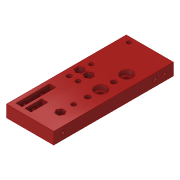
# Autodesk Inventor part: Coupler lift short left
Saved by Autodesk Inventor 2020 (Build 240168000, 168)
## iProperties
Created: 2019-10-02
Part Number: Coupler lift short left
Material: Generic
Document SubType Name: Modeling
Designer: ball
Density: 1 g/cm^3
Appearance: Default
Author: ball
Autodesk Inventor part; units mm, degrees
ref_plane "YZ Plane" through (0, 0, 0) normal (1, 0, 0) x (0, 1, 0)
sketch "Sketch1" plane through (0, 0, 0) normal (0, 1, 0) x (-1, 0, 0)
  line L0 (0, 0) -> (35.5, 0)
  line L1 (35.5, 0) -> (35.5, -90)
  line L2 (35.5, -90) -> (0, -90)
  line L3 (0, -90) -> (0, 0)
  dimension "d0" = 35.5
  dimension "d1" = 90
  constraints: 8 end point, 2 parallel, 1 horizontal, 1 perpendicular
  measures "d0" distance of L1.end L2.end
  measures "d1" distance of L0.end L1.end
extrude "BlockShape" add sketch "Sketch1" along normal blind 9
sketch "Sketch3" plane through (0, 0, 0) normal (0, -1, 0) x (1, 0, 0)
  circle A0 centre (-10, -25) radius 3.25 construction
  line L0 (0, 0) -> (-35.5, 0) projected
  line L1 (-35.5, 0) -> (-35.5, -90) projected
  line L2 (-11.6286, -27.8125) -> (-13.25, -24.9958)
  line L3 (-13.25, -24.9958) -> (-11.6214, -22.1833)
  line L4 (-11.6214, -22.1833) -> (-8.3714, -22.1875)
  line L5 (-8.3714, -22.1875) -> (-6.75, -25.0042)
  line L6 (-6.75, -25.0042) -> (-8.3786, -27.8167)
  line L7 (-8.3786, -27.8167) -> (-11.6286, -27.8125)
  line L8 (0, -90) -> (0, 0) projected
  dimension "d15" = 6.5
  dimension "d16" = 25
  dimension "d26" = 10
  constraints: 12 end point, 1 coincident, 16 other
  measures "d16" distance from line of L0 point (-10, -25)
  measures "d26" distance from line of L8 point (-10, -25)
extrude "SlideMountingNutWell1" cut sketch "Sketch3" against normal blind 5
sketch "Sketch5" plane through (0, 9, 0) normal (0, 1, 0) x (1, 0, 0)
  line L0 (0, 0) -> (0, 90) projected
  line L1 (-35.5, 0) -> (0, 0) projected
  circle A0 centre (-10, 25) radius 1.7
  circle A1 centre (-10, 15) radius 1.7
  dimension "d36" = 3.4
  dimension "d37" = 25
  dimension "d137" = 3.4
  dimension "d138" = 15
  constraints: 2 centre point
  measures "d36" diameter of A0
  measures "d37" distance from line of L1 A0.centre
  measures "d137" diameter of A1
  measures "d138" distance from line of L1 A1.centre
extrude "SlideMountingHoles" cut sketch "Sketch5" against normal through all
sketch "Sketch6" plane through (0, 9, 0) normal (0, 1, 0) x (1, 0, 0)
  line L0 (-32.5, 4) -> (-27.7502, 4)
  line L1 (-27.7502, 4) -> (-27.7502, 29.4)
  line L2 (-27.7502, 29.4) -> (-32.5, 29.4)
  line L3 (-32.5, 29.4) -> (-32.5, 4)
  line L4 (-35.5, 0) -> (0, 0) projected
  line L5 (-35.5, 90) -> (-35.5, 0) projected
  line L6 (-25.7502, 4) -> (-21.0002, 4)
  line L7 (-21.0002, 4) -> (-21.0002, 16.7)
  line L8 (-21.0002, 16.7) -> (-25.7502, 16.7)
  line L9 (-25.7502, 16.7) -> (-25.7502, 4)
  line L10 (0, 0) -> (0, 90) construction
  line L11 (-35.5, 90) -> (0, 90) projected
  line L12 (0, 0) -> (-20, 0) construction
  line L13 (-20, 0) -> (-20, 90) construction
  line L14 (-20, 90) -> (0, 90) construction
  line L15 (0, 90) -> (0, 0)
  circle A0 centre (-23.3752, 41.7) radius 1.7
  circle A1 centre (-30.125, 41.7) radius 1.7
  circle A2 centre (-30.125, 49.7) radius 1.7
  circle A3 centre (-23.3752, 49.7) radius 1.7
  dimension "d43" = 4.7498
  dimension "d44" = 25.4
  dimension "d45" = 4
  dimension "d46" = 3
  dimension "d47" = 4.75
  dimension "d48" = 2
  dimension "d49" = 20
  dimension "d50" = 3.4
  dimension "d90" = 3.4
  dimension "d91" = 5.375
  dimension "d92" = 3.4
  dimension "d93" = 8
  dimension "d94" = 3.4
  dimension "d99" = 40.3
  constraints: 24 end point, 6 parallel, 4 centre point, 3 horizontal, 3 perpendicular, 1 point on line
  measures "d43" distance of L2.end L1.end
  measures "d44" distance of L1.end L0.end
  measures "d45" distance between parallel lines of L4 L0
  measures "d46" distance between parallel lines of L5 L3
  measures "d47" distance of L8.end L7.end
  measures "d48" distance between parallel lines of L9 L1
  measures "d49" distance of L13.end L14.end
  measures "d50" diameter of A0
  measures "d90" diameter of A1
  measures "d91" distance from line of L5 A1.centre
  measures "d92" diameter of A2
  measures "d93" distance of A2.centre A1.centre
  measures "d94" diameter of A3
  measures "d99" distance from line of L11 A2.centre
extrude "Shape" cut sketch "Sketch6" against normal through all contours L3 L2 L1 L0 | L9 L8 L7 L6 | A0 | A1 | A2 | A3
sketch "Sketch7" plane through (0, 0, 0) normal (0, -1, 0) x (1, 0, 0)
  circle A0 centre (-23.3752, -41.7) radius 1.7 projected
  circle A1 centre (-23.3752, -41.7) radius 3.25 construction
  line L0 (-23.3752, -38.45) -> (-20.5606, -40.075)
  line L1 (-20.5606, -40.075) -> (-20.5606, -43.325)
  line L2 (-20.5606, -43.325) -> (-23.3752, -44.95)
  line L3 (-23.3752, -44.95) -> (-26.1898, -43.325)
  line L4 (-26.1898, -43.325) -> (-26.1898, -40.075)
  line L5 (-26.1898, -40.075) -> (-23.3752, -38.45)
  line L6 (0, 0) -> (-35.5, 0) projected
  circle A2 centre (-30.125, -41.7) radius 3.25 construction
  line L7 (-35.5, 0) -> (-35.5, -90) projected
  line L8 (-30.1645, -44.9498) -> (-32.9591, -43.2907)
  line L9 (-32.9591, -43.2907) -> (-32.9196, -40.0409)
  line L10 (-32.9196, -40.0409) -> (-30.0855, -38.4502)
  line L11 (-30.0855, -38.4502) -> (-27.2909, -40.1093)
  line L12 (-27.2909, -40.1093) -> (-27.3304, -43.3591)
  line L13 (-27.3304, -43.3591) -> (-30.1645, -44.9498)
  dimension "d88" = 6.5
  dimension "d54" = 6.5
  dimension "d87" = 41.7
  dimension "d89" = 5.375
  constraints: 24 end point, 3 coincident, 1 centre point, 17 other
  measures "d54" diameter of A1
  measures "d87" distance from line of L6 A1.centre
  measures "d89" distance from line of L7 point (-30.125, -41.7)
extrude "TensionNutWells1" cut sketch "Sketch7" against normal blind 5
sketch "Sketch8" plane through (-35.5, 0, -90) normal (-1, 0, 0) x (0, 0, 1)
  circle A0 centre (79.65, 4.5) radius 1.4605
  line L0 (0, 9) -> (90, 9) projected
  line L1 (90, 0) -> (90, 9) projected
  circle A1 centre (66.95, 4.5) radius 1.4605
  dimension "d57" = 2.921
  dimension "d58" = 4.5
  dimension "d59" = 10.35
  dimension "d103" = 2.921
  dimension "d104" = 4.5
  dimension "d105" = 12.7
  constraints: 2 centre point
  measures "d57" diameter of A0
  measures "d58" distance from line of L0 A0.centre
  measures "d59" distance from line of L1 A0.centre
  measures "d103" diameter of A1
  measures "d104" distance from line of L0 A1.centre
  measures "d105" distance of A0.centre A1.centre
hole "PulleyMountingHoles" at (-35.5, 4.5, -10.35) at (-35.5, 4.5, -23.05) direction (1, 0, 0) diameter 2.921 depth 22.5 counterbore diameter 3.4 counterbore depth 1.5
sketch "Sketch9" plane through (-21.0002, 9, -16.7) normal (-1, 0, 0) x (0, 0, 1)
  circle A0 centre (6.35, -4.5) radius 1.4605 projected
  circle A1 centre (6.35, -4.5) radius 2.54
  point P0 (16.7, -9)
  dimension "d67" = 5.08
  constraints: 1 centre point, 1 coincident
  measures "d67" diameter of A1
extrude "PulleyStandoff1" add sketch "Sketch9" along normal blind 0.2032
sketch "Sketch10" plane through (-27.7502, 9, -29.4) normal (-1, 0, 0) x (0, 0, 1)
  circle A0 centre (6.35, -4.5) radius 1.7 projected
  circle A1 centre (6.35, -4.5) radius 2.54
  circle A2 centre (19.05, -4.5) radius 2.54 projected
  circle A3 centre (19.05, -4.5) radius 2.54
  circle A4 centre (19.05, -4.5) radius 1.7
  point P0 (29.4, -9)
  dimension "d70" = 5.08
  dimension "d106" = 3.4
  constraints: 3 centre point, 3 coincident
  measures "d70" diameter of A1
  measures "d106" diameter of A4
extrude "PulleyStandoff3" add sketch "Sketch10" along normal blind 0.2032
sketch "Sketch11" plane through (-25.7502, 9, -4) normal (1, 0, 0) x (0, 0, -1)
  circle A0 centre (6.35, -4.5) radius 1.7 projected
  circle A1 centre (6.35, -4.5) radius 2.54
  point P0 (-4, -9)
  dimension "d73" = 5.08
  constraints: 1 centre point, 1 coincident
  measures "d73" diameter of A1
extrude "PulleyStandoff2" add sketch "Sketch11" along normal blind 0.2032
sketch "Sketch12" plane through (-32.5, 9, -4) normal (1, 0, 0) x (0, 0, -1)
  circle A0 centre (6.35, -4.5) radius 1.7 projected
  circle A1 centre (6.35, -4.5) radius 2.54
  circle A2 centre (19.05, -4.5) radius 1.4605 projected
  circle A3 centre (19.05, -4.5) radius 2.54
  circle A4 centre (19.05, -4.5) radius 1.7
  point P0 (-4, -9)
  dimension "d76" = 5.08
  dimension "d107" = 5.08
  dimension "d108" = 3.4
  constraints: 3 centre point, 3 coincident
  measures "d76" diameter of A1
  measures "d107" diameter of A3
  measures "d108" diameter of A4
extrude "PulleyStandof4" add sketch "Sketch12" along normal blind 0.2032 contours A1 | A3
sketch "Sketch14" plane through (0, 0, -90) normal (0, 0, -1) x (-1, 0, 0)
  circle A0 centre (18, 4.5) radius 2.25
  line L0 (35.5, 0) -> (0, 0) projected
  line L1 (0, 0) -> (0, 9) projected
  dimension "d82" = 4.5
  dimension "d83" = 4.5
  dimension "d84" = 18
  constraints: 1 centre point
  measures "d82" diameter of A0
  measures "d83" distance from line of L0 A0.centre
  measures "d84" distance from line of L1 A0.centre
extrude "4mmShaft" cut sketch "Sketch14" against normal blind 41
sketch "Sketch15" plane through (0, 9, 0) normal (0, 1, 0) x (1, 0, 0)
  circle A0 centre (-30.125, 49.7) radius 1.7 projected
  circle A1 centre (-30.125, 49.7) radius 3.25 construction
  circle A2 centre (-23.3752, 49.7) radius 1.7 projected
  circle A3 centre (-23.3752, 49.7) radius 3.25 construction
  line L0 (-30.125, 52.95) -> (-27.3104, 51.325)
  line L1 (-27.3104, 51.325) -> (-27.3104, 48.075)
  line L2 (-27.3104, 48.075) -> (-30.125, 46.45)
  line L3 (-30.125, 46.45) -> (-32.9396, 48.075)
  line L4 (-32.9396, 48.075) -> (-32.9396, 51.325)
  line L5 (-32.9396, 51.325) -> (-30.125, 52.95)
  line L6 (-23.3752, 52.95) -> (-20.5606, 51.325)
  line L7 (-20.5606, 51.325) -> (-20.5606, 48.075)
  line L8 (-20.5606, 48.075) -> (-23.3752, 46.45)
  line L9 (-23.3752, 46.45) -> (-26.1898, 48.075)
  line L10 (-26.1898, 48.075) -> (-26.1898, 51.325)
  line L11 (-26.1898, 51.325) -> (-23.3752, 52.95)
  point P0 (0, 0)
  dimension "d95" = 6.5
  dimension "d96" = 6.5
  constraints: 24 end point, 4 coincident, 2 vertical alignment, 30 other
extrude "TensionNutWells2" cut sketch "Sketch15" against normal blind 5
ref_plane "PulleyMidPlane1" through (-30.1251, 9, -4) normal (1, 0, 0) x (0, 0, -1)
ref_plane "PulleyMidPlane2" through (-23.3752, 9, -4) normal (1, 0, 0) x (0, 0, -1)
sketch "Sketch20" plane through (0, 9, 0) normal (0, 1, 0) x (1, 0, 0)
  circle A0 centre (-29.5, 86) radius 1.524
  circle A1 centre (-29.5, 57.7) radius 1.524
  line L0 (-35.5, 90) -> (-35.5, 0) projected
  line L1 (0, 90) -> (-35.5, 90) projected
  circle A2 centre (-30.125, 49.7) radius 1.7 projected
  point P0 (0, 0)
  dimension "d129" = 3.048
  dimension "d130" = 3.048
  dimension "d131" = 6
  dimension "d132" = 4
  dimension "d133" = 6
  dimension "d134" = 8
  constraints: 2 centre point
  measures "d129" diameter of A0
  measures "d130" diameter of A1
  measures "d131" distance from line of L0 A0.centre
  measures "d132" distance from line of L1 A0.centre
  measures "d133" distance from line of L0 A1.centre
  measures "d134" vertical distance of A2.centre A1.centre
extrude "TieWrapHoles" cut sketch "Sketch20" against normal through all contours A0 | A1
sketch "Sketch21" plane through (0, 9, 0) normal (0, 1, 0) x (1, 0, 0)
  circle A0 centre (-10, 15) radius 1.7 construction
  circle A1 centre (-10, 15) radius 3.25 construction
  line L0 (-6.75, 15) -> (-8.375, 12.1854)
  line L1 (-8.375, 12.1854) -> (-11.625, 12.1854)
  line L2 (-11.625, 12.1854) -> (-13.25, 15)
  line L3 (-13.25, 15) -> (-11.625, 17.8146)
  line L4 (-11.625, 17.8146) -> (-8.375, 17.8146)
  line L5 (-8.375, 17.8146) -> (-6.75, 15)
  point P0 (0, 0)
  dimension "d139" = 6.5
  constraints: 12 end point, 2 coincident, 1 horizontal alignment, 15 other
extrude "SlideMountingNutWell2" cut sketch "Sketch21" against normal blind 5
sketch "Sketch22" plane through (0, 0, 0) normal (0, -1, 0) x (1, 0, 0)
  circle A0 centre (-9.525, -35) radius 1.9304 construction
  circle A1 centre (-9.525, -54.558) radius 1.9304 construction
  circle A2 centre (-10, -25) radius 1.7 construction
  line L0 (0, -90) -> (0, 0) construction
  dimension "d142" = 3.8608
  dimension "d143" = 3.8608
  dimension "d144" = 19.558
  dimension "d145" = 9.525
  dimension "d146" = 10
  constraints: 2 centre point
  measures "d142" diameter of A0
  measures "d143" diameter of A1
  measures "d144" distance of A1.centre A0.centre
  measures "d145" distance from line of A0.centre L0
  measures "d146" vertical distance of A0.centre A2.centre
hole "XRrailMountingHoles1" at (-9.525, 0, -54.558) at (-9.525, 0, -35) direction (0, 1, 0) diameter 3.8608 end through all counterbore diameter 8.89 counterbore depth 3.048
sketch "Sketch23" plane through (0, 9, 0) normal (0, 1, 0) x (1, 0, 0)
  circle A0 centre (-9.525, 44.779) radius 1.9304 construction
  circle A1 centre (-9.525, 64.337) radius 1.9304 construction
  circle A2 centre (-9.525, 35) radius 1.9304 projected
  line L0 (0, 0) -> (0, 90) projected
  dimension "d154" = 3.8608
  dimension "d155" = 3.8608
  dimension "d156" = 19.558
  dimension "d157" = 9.779
  dimension "d158" = 9.525
  constraints: 2 centre point
  measures "d154" diameter of A0
  measures "d155" diameter of A1
  measures "d156" distance of A1.centre A0.centre
  measures "d157" distance of A2.centre A0.centre
  measures "d158" distance from line of L0 A0.centre
hole "XRrailMountingHoles2" at (-9.525, 9, -44.779) at (-9.525, 9, -64.337) direction (0, -1, 0) diameter 3.8608 end through all counterbore diameter 8.89 counterbore depth 3.048
sketch "Sketch25" plane through (0, 0, 0) normal (1, 0, 0) x (0, 0, -1)
  circle A0 centre (6.65, 4.5) radius 1.45
  line L0 (90, 0) -> (0, 0) construction
  line L1 (0, 9) -> (90, 9) construction
  line L2 (13.3, 4) -> (13.3, 0) construction
  line L3 (0, 0) -> (0, 9) construction
  line L4 (66.2674, 5.952) -> (62.4066, 5.952) construction
  line L5 (59.892, 9) -> (68.782, 9) construction
  line L6 (68.782, 5.952) -> (59.892, 5.952) construction
  line L7 (90, 0) -> (90, 9) construction
  circle A1 centre (75.8547, 4.5) radius 1.45
  circle A2 centre (82.9273, 4.5) radius 1.45
  dimension "d178" = 2.9
  dimension "d179" = 9
  dimension "d180" = 4.5
  dimension "d181" = 13.3
  dimension "d182" = 6.65
  dimension "d183" = 21.218
  dimension "d184" = 2.9
  dimension "d185" = 2.9
  dimension "d186" = 4.5
  dimension "d187" = 4.5
  dimension "d188" = 7.0727
  dimension "d189" = 7.0727
  constraints: 3 centre point
  measures "d178" diameter of A0
  measures "d179" distance between parallel lines of L0 L1
  measures "d180" distance from line of L0 A0.centre
  measures "d181" distance between parallel lines of L3 L2
  measures "d182" distance from line of L3 A0.centre
  measures "d183" distance from line of L7 L6.start
  measures "d184" diameter of A1
  measures "d185" diameter of A2
  measures "d186" distance from line of L0 A1.centre
  measures "d187" distance from line of L0 A2.centre
  measures "d188" distance from line of A2.centre L7
  measures "d189" distance of A1.centre A2.centre
extrude "NonPulleySideHoles" cut sketch "Sketch25" against normal blind 13
sketch "Sketch26" plane through (-35.5, 0, -90) normal (-1, 0, 0) x (0, 0, 1)
  line L0 (60.6, 9) -> (60.6, 0) construction
  line L1 (51.5498, 0) -> (51.5498, 5) construction
  line L2 (33.824, 0) -> (30.776, 0) construction
  line L3 (5.524, 0) -> (2.476, 0) construction
  circle A0 centre (56.0749, 4.5) radius 1.45
  circle A1 centre (24.463, 4.5) radius 1.45
  line L4 (30.776, 9) -> (30.776, 0) construction
  line L5 (5.524, 9) -> (5.524, 0) construction
  line L6 (0, 9) -> (90, 9) projected
  circle A2 centre (18.15, 4.5) radius 1.45
  circle A3 centre (11.837, 4.5) radius 1.45
  point P0 (90, 0)
  dimension "d192" = 2.9
  dimension "d193" = 2.9
  dimension "d196" = 25.252
  dimension "d197" = 6.313
  dimension "d198" = 4.5
  dimension "d199" = 4.5
  dimension "d202" = 6.313
  dimension "d207" = 9.0502
  dimension "d208" = 4.5251
  constraints: 4 centre point, 1 horizontal, 4 other
  measures "d192" diameter of A0
  measures "d193" diameter of A1
  measures "d196" distance between parallel lines of L5 L4
  measures "d197" distance from line of L4 A1.centre
  measures "d198" distance from line of L6 A0.centre
  measures "d199" distance from line of L6 A1.centre
  measures "d202" distance of A1.centre A2.centre
  measures "d207" distance between parallel lines of L1 L0
  measures "d208" distance from line of L0 A0.centre
extrude "PulleySideHoles" cut sketch "Sketch26" against normal blind 13
equation "\"d133\" = d131"
equation "\"d157\" = 0.5 * d156"
equation "\"d158\" = d145"
equation "\"d180\" = 0.5 * d179"
equation "\"d182\" = 0.5 * d181"
equation "\"d186\" = d180"
equation "\"d187\" = d180"
equation "\"d188\" = 0.333333 * d183"
equation "\"d189\" = d188"
equation "\"d197\" = 0.25 * d196"
equation "\"d198\" = d180"
equation "\"d199\" = d180"
equation "\"d202\" = d197"
equation "\"d208\" = 0.5 * d207"
body "Solid1"
